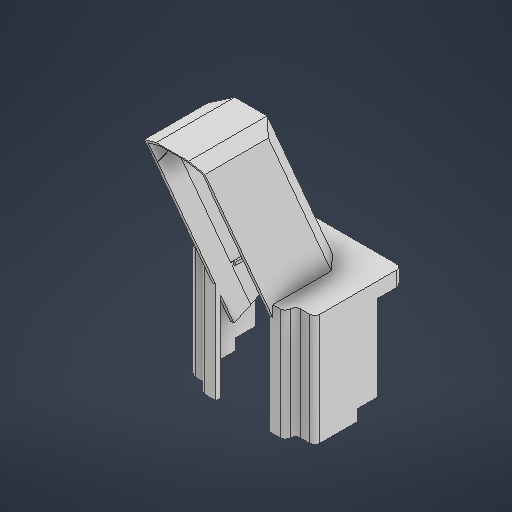
# Autodesk Inventor part: Cover^2 No magnets
Saved by Autodesk Inventor 2025 (Build 290162000, 162)
## iProperties
Created: 2025-02-14
Part Number: Cover^2 No magnets
Material: Generic
Document SubType Name: Modeling
Designer: mayhe
Density: 1 g/cm^3
Appearance: Default
Author: mayhe
Autodesk Inventor part; units mm, degrees
ref_plane "YZ Plane" through (0, 0, 0) normal (1, 0, 0) x (0, 1, 0)
ref_plane "XZ Plane" through (0, 0, 0) normal (0, 1, 0) x (-1, 0, 0)
ref_plane "XY Plane" through (0, 0, 0) normal (0, 0, 1) x (1, 0, 0)
sketch "Sketch1" plane through (0, 0, 0) normal (0, 1, 0) x (-1, 0, 0)
  line L0 (58.5, -37.5625) -> (-58.5, -37.5625)
  line L1 (-58.5, -37.5625) -> (-58.5, 37.5625)
  line L2 (-58.5, 37.5625) -> (58.5, 37.5625)
  line L3 (58.5, 37.5625) -> (58.5, -37.5625)
  line L4 (58.5, -37.5625) -> (-58.5, 37.5625) construction
  line L5 (-58.5, -37.5625) -> (58.5, 37.5625) construction
  line L6 (-61.5, -40.5625) -> (61.5, -40.5625)
  line L7 (61.5, -40.5625) -> (61.5, 37.5625)
  line L8 (-61.5, 37.5625) -> (-61.5, -40.5625)
  line L9 (-58.5, 37.5625) -> (-61.5, 37.5625)
  line L10 (58.5, 37.5625) -> (61.5, 37.5625)
  line L11 (-25, 25.0625) -> (25, 25.0625)
  line L12 (25, 25.0625) -> (25, 50.0625)
  line L13 (25, 50.0625) -> (-25, 50.0625)
  line L14 (-25, 50.0625) -> (-25, 25.0625)
  line L15 (-25, 25.0625) -> (25, 50.0625) construction
  line L16 (25, 25.0625) -> (-25, 50.0625) construction
  line L17 (61.5, 37.5625) -> (26.5, 37.5625)
  line L18 (26.5, 37.5625) -> (26.5, 52.5625)
  line L19 (-61.5, 37.5625) -> (-26.5, 37.5625)
  line L20 (-26.5, 37.5625) -> (-26.5, 52.5625)
  line L21 (25, 25.0625) -> (-25, 25.0625)
  line L22 (-25, 25.0625) -> (-25, 10.0625)
  line L23 (-25, 10.0625) -> (25, 10.0625)
  line L24 (25, 10.0625) -> (25, 25.0625)
  circle A0 centre (0, 10.0625) radius 25
  line L25 (61.5, 37.5625) -> (61.5, 45.5625)
  line L26 (61.5, 45.5625) -> (42.25, 45.5625)
  line L27 (42.25, 45.5625) -> (42.25, 55.5625)
  line L28 (42.25, 55.5625) -> (26.5, 55.5625)
  line L29 (26.5, 55.5625) -> (26.5, 52.5625)
  line L30 (-26.5, 52.5625) -> (-26.5, 55.5625)
  line L31 (-26.5, 55.5625) -> (-42.25, 55.5625)
  line L32 (-42.25, 55.5625) -> (-42.25, 45.5625)
  line L33 (-42.25, 45.5625) -> (-61.5, 45.5625)
  line L34 (-61.5, 45.5625) -> (-61.5, 37.5625)
  point P0 (0, 0)
  point P1 (0, 37.5625)
  point P2 (25, 37.5625)
  point P3 (-25, 37.5625)
  point P4 (-26.5, 37.5625)
  point P5 (26.5, 37.5625)
  point P6 (58.5, 37.5625)
  dimension "d1" = 75.125
  dimension "d2" = 3
  dimension "d10" = 50
  dimension "d11" = 25
  dimension "d23" = 3
  dimension "d33" = 50
  dimension "d34" = 15
  dimension "d65" = 8
  dimension "d67" = 10
  dimension "d69" = 15.75
  dimension "d70" = 10
  dimension "d71" = 19.25
  dimension "d72" = 8
  dimension "d85" = 15.75
  dimension "d86" = 19.25
  constraints: 70 end point, 14 perpendicular, 7 parallel, 6 horizontal, 6 midpoint, 1 point on line, 1 vertical, 3 other
  measures "d1" distance between parallel lines of L2 L0
  measures "d2" distance between parallel lines of L0 L6
  measures "d10" distance of L13.end L12.end
  measures "d11" distance of L12.end L11.end
  measures "d23" distance between parallel lines of L3 L7
  measures "d33" distance of L23.end L22.end
  measures "d34" distance of L22.end L21.end
  measures "d65" distance of L7.end L25.end
  measures "d67" distance of L26.end L27.end
  measures "d69" distance of L30.end L31.end
  measures "d70" distance of L31.end L32.end
  measures "d71" distance of L32.end L33.end
  measures "d72" distance of L33.end L8.start
  measures "d85" distance of L27.end L28.end
  measures "d86" distance of L25.end L26.end
extrude "Extrusion1" add sketch "Sketch1" along normal blind 3 contours L3 L10 L7 L6 L8 L9 L1 L0 | L0 L1 L2 L14 L22 A0 L24 L12 L3 | L2 L18 L29 L28 L27 L26 L25 L10 | L9 L34 L33 L32 L31 L30 L20 L2
sketch "Sketch2" plane through (0, 0, 0) normal (0, -1, 0) x (1, 0, 0)
  line L0 (-59.5, 43.5625) -> (-59.5, 20.5625)
  line L1 (-59.5, 20.5625) -> (-61.5, 20.5625)
  line L2 (-61.5, 20.5625) -> (-61.5, 45.5625)
  line L3 (0, 0) -> (0, 37.5625)
  line L4 (59.5, 20.5625) -> (61.5, 20.5625)
  line L5 (-42.25, 55.5625) -> (-26.5, 55.5625)
  line L6 (-26.5, 55.5625) -> (-26.5, 50.5625)
  line L7 (-26.5, 50.5625) -> (-40.25, 50.5625)
  line L8 (-42.25, 45.5625) -> (-61.5, 45.5625)
  line L9 (-59.5, 43.5625) -> (-40.25, 43.5625)
  line L10 (-40.25, 43.5625) -> (-40.25, 50.5625)
  line L11 (-42.25, 45.5625) -> (-42.25, 55.5625) projected
  line L12 (-42.25, 55.5625) -> (-42.25, 45.5625)
  line L13 (59.5, 43.5625) -> (59.5, 20.5625)
  line L14 (59.5, 20.5625) -> (61.5, 20.5625)
  line L15 (61.5, 20.5625) -> (61.5, 45.5625)
  line L16 (42.25, 55.5625) -> (26.5, 55.5625)
  line L17 (26.5, 55.5625) -> (26.5, 50.5625)
  line L18 (26.5, 50.5625) -> (40.25, 50.5625)
  line L19 (42.25, 45.5625) -> (61.5, 45.5625)
  line L20 (59.5, 43.5625) -> (40.25, 43.5625)
  line L21 (40.25, 43.5625) -> (40.25, 50.5625)
  line L22 (42.25, 45.5625) -> (42.25, 55.5625)
  line L23 (42.25, 55.5625) -> (42.25, 45.5625)
  point P0 (0, 25.0625)
  point P1 (-59.5, 53.5625)
  dimension "d6" = 2
  dimension "d27" = 5
  dimension "d76" = 2
  dimension "d77" = 2
  dimension "d78" = 19.25
  dimension "d79" = 19.25
  dimension "d80" = 25
  constraints: 46 end point, 11 symmetric about line, 4 perpendicular, 2 parallel, 1 coincident, 1 collinear, 1 horizontal, 1 vertical, 1 vertical alignment
  measures "d6" distance of L0.end L1.end
  measures "d27" distance of L5.end L6.end
  measures "d76" distance between parallel lines of L11 L10
  measures "d77" distance between parallel lines of L9 L8
  measures "d78" distance of L8.start L2.end
  measures "d79" distance of L0.start L9.end
  measures "d80" distance of L1.end L2.end
extrude "Extrusion2" add sketch "Sketch2" along normal blind 107.5
sketch "Sketch3" plane through (0, 0, 0) normal (0, -1, 0) x (1, 0, 0)
  line L0 (61.5, -40.5625) -> (-61.5, -40.5625) projected
  line L1 (-61.5, -40.5625) -> (61.5, -40.5625)
  line L2 (61.5, -40.5625) -> (61.5, -16.5625)
  line L3 (61.5, -16.5625) -> (56, -16.5625)
  line L4 (56, -16.5625) -> (56, -37.5625)
  line L5 (-61.5, -16.5625) -> (-61.5, -40.5625)
  line L6 (-61.5, -16.5625) -> (-56, -16.5625)
  line L7 (-56, -16.5625) -> (-56, -37.5625)
  line L8 (-56, -37.5625) -> (56, -37.5625)
  line L9 (-59.5, 20.4625) -> (-59.5, -16.5625)
  line L10 (-59.5, -16.5625) -> (-61.5, -16.5625)
  line L11 (61.5, 20.5625) -> (61.5, 55.5625) projected
  line L12 (61.5, 20.5625) -> (59.5, 20.5625)
  line L13 (59.5, 20.5625) -> (59.5, -16.5625)
  line L14 (59.5, -16.5625) -> (61.5, -16.5625)
  line L15 (61.5, -16.5625) -> (61.5, 20.5625)
  line L16 (-61.5, -40.5625) -> (-61.5, 45.5625) projected
  line L17 (-61.5, 20.5625) -> (-61.5, -16.5625)
  line L18 (-61.5, -16.5625) -> (-61.5, -40.5625)
  line L19 (-61.5, 20.5625) -> (-59.5, 20.5625) projected
  line L20 (-61.5, 20.5625) -> (-59.5, 20.5625)
  line L21 (-59.5, 20.5625) -> (-59.5, 20.4625)
  point P0 (0, 0)
  dimension "d12" = 24
  dimension "d13" = 5.5
  dimension "d15" = 90
  dimension "d20" = 5.5
  dimension "d22" = 3
  dimension "d31" = 2
  dimension "d32" = 2
  constraints: 36 end point, 8 perpendicular, 3 collinear, 3 horizontal, 3 point on line, 2 parallel
  measures "d12" distance of L0.start L2.end
  measures "d13" distance of L2.end L3.end
  measures "d15" angle of L4 L3
  measures "d20" distance of L5.start L6.end
  measures "d22" distance between parallel lines of L0 L8
  measures "d31" distance of L9.end L10.end
  measures "d32" distance of L14.end L13.end
extrude "Extrusion3" add sketch "Sketch3" along normal blind 12
fillet "Fillet1" radius 5 16 edges at (56, -6, -37.5625) (-56, -6, -37.5625) (61.5, -4.5, -40.5625) (-61.5, -4.5, -40.5625) (61.5, -52.25, 45.5625) (42.25, -52.25, 45.5625) (42.25, -52.25, 55.5625) (-42.25, -52.25, 55.5625) (-61.5, -52.25, 45.5625) (-42.25, -52.25, 45.5625) (-59.5, -53.75, 43.5625) (-40.25, -53.75, 50.5625) (-40.25, -53.75, 43.5625) (40.25, -53.75, 50.5625) (40.25, -53.75, 43.5625) (59.5, -53.75, 43.5625)
chamfer "Chamfer1" distance 3.5 angle 45 2 edges at (-56, -6, -16.5625) (56, -6, -16.5625)
ref_plane "Work Plane1" through (-42.25, 3, 55.5625) normal (0, 0.9187912, 0.3947439) x (1, 0, 0)
sketch "Sketch4" plane through (-42.25, 3, 55.5625) normal (0, 0.9187912, 0.3947439) x (1, 0, 0)
  line L0 (15.25, 63.1227) -> (69.25, 63.1227)
  line L1 (69.25, 63.1227) -> (69.25, 13.7819)
  ellipse E0 centre (42.25, 41.805) end of major axis (67.25, 41.805) minor radius 22.9698 (67.25, 41.805) -> (17.25, 41.805) ccw
  line L2 (42.25, 41.805) -> (15.25, 63.1227) construction
  line L3 (42.25, 41.805) -> (69.25, 63.1227) construction
  line L4 (12.25, 53.6373) -> (12.25, -4.3627)
  line L5 (72.25, -4.3627) -> (72.25, 53.6373)
  line L6 (72.25, 53.6373) -> (12.25, 53.6373)
  line L7 (15.75, 13.7819) -> (15.25, 13.7819)
  line L8 (15.75, 13.7819) -> (15.75, -4.3627)
  line L9 (67.75, 16.5382) -> (67.75, 0)
  line L10 (69.25, 13.7819) -> (68.75, 13.7819)
  line L11 (68.75, 13.7819) -> (68.75, -4.3627)
  line L12 (12.25, -4.3627) -> (15.75, -4.3627)
  line L13 (68.75, -4.3627) -> (72.25, -4.3627)
  line L14 (15.25, 13.7819) -> (15.25, 63.1227)
  line L15 (12.25, 53.6373) -> (12.25, 67.1227)
  line L16 (12.25, 67.1227) -> (72.25, 67.1227)
  line L17 (72.25, 67.1227) -> (72.25, 53.6373)
  point P0 (42.25, 49.0766)
  point P1 (15.25, 53.6373)
  point P2 (69.25, 53.6373)
  point P3 (42.25, 53.6373)
  point P4 (42.25, 64.7748)
  point P5 (42.25, 67.1227)
  point P6 (42.25, 63.1227)
  dimension "d36" = 54
  dimension "d39" = 58
  dimension "d40" = 3.5
  dimension "d41" = 60
  dimension "d47" = 4
  dimension "d57" = 3
  constraints: 32 end point, 3 midpoint, 3 point on line, 2 vertical alignment, 11 other
  measures "d36" distance of L0.start L0.end
  measures "d39" distance between parallel lines of L6 L12
  measures "d40" distance between parallel lines of L8 L4
  measures "d41" distance of L5.start L4.end
  measures "d47" distance between parallel lines of L0 L16
  measures "d57" distance between parallel lines of L14 L4
extrude "Extrusion4" add sketch "Sketch4" along normal blind 135 and the other way blind 55.8 contours L14 L6 L15 L16 L17 L1 L0 E0 | E0 L0 | L14 L7 L8 L12 L4 L6 | L6 L5 L13 L11 L10 L1
chamfer "Chamfer3" distance 14 angle 45 4 edges at (-30, 78.2665, 14.8441) (30, 78.2665, 14.8441) (-27, 77.4771, 18.8585) (27, 77.4771, 18.8585)
sketch "Sketch9" plane through (0, -12, 0) normal (0, -1, 0) x (1, 0, 0)
  line L0 (0, 0) -> (0, 50)
  line L1 (-61.5, 20.5625) -> (-59.5, 20.5625) projected
  line L2 (-59.5, -16.5625) -> (-59.5, 20.5625) projected
  line L3 (-61.5, 20.5625) -> (-59.5, 20.5625)
  line L4 (-59.5, 20.5625) -> (-59.5, -16.5625)
  line L5 (-59.5, -16.5625) -> (-61.5, -16.5625)
  line L6 (-61.5, -16.5625) -> (-61.5, 20.5625)
  line L7 (61.5, 20.5625) -> (59.5, 20.5625)
  line L8 (59.5, -16.5625) -> (59.5, 20.5625)
  line L9 (61.5, 20.5625) -> (59.5, 20.5625)
  line L10 (59.5, 20.5625) -> (59.5, -16.5625)
  line L11 (59.5, -16.5625) -> (61.5, -16.5625)
  line L12 (61.5, -16.5625) -> (61.5, 20.5625)
  dimension "d92" = 50
  constraints: 22 end point, 5 symmetric about line, 2 parallel, 1 horizontal, 1 perpendicular, 1 vertical
  measures "d92" distance of L0.start L0.end
extrude "Extrusion8" add sketch "Sketch9" along normal blind 95.5
sketch "Sketch10" plane through (0, -107.5, 0) normal (0, -1, 0) x (1, 0, 0)
  line L0 (-59.5, -16.5625) -> (-56, -20.0625) projected
  line L1 (-61.5, 40.5625) -> (-61.5, -16.5625) projected
  line L2 (-59.5, -16.5625) -> (-61.5, -16.5625)
  line L3 (-61.5, -16.5625) -> (-61.5, 3.4375)
  line L4 (-61.5, 3.4375) -> (-59.5, 3.4375)
  line L5 (-59.5, 3.4375) -> (-59.5, -16.5625)
  line L6 (0, 0) -> (0, 17.4625)
  line L7 (59.5, -16.5625) -> (56, -20.0625)
  line L8 (61.5, 40.5625) -> (61.5, -16.5625)
  line L9 (59.5, -16.5625) -> (61.5, -16.5625)
  line L10 (61.5, -16.5625) -> (61.5, 3.4375)
  line L11 (61.5, 3.4375) -> (59.5, 3.4375)
  line L12 (59.5, 3.4375) -> (59.5, -16.5625)
  dimension "d93" = 20
  constraints: 22 end point, 7 symmetric about line, 2 parallel, 2 point on line, 1 horizontal, 1 perpendicular, 1 vertical
  measures "d93" distance of L2.end L3.end
extrude "Extrusion9" cut sketch "Sketch10" against normal blind 11
ref_plane "Work Plane5" through (-30, 64.798, 86.8613) normal (0, 0, 1) x (1, 0, 0)
sketch "Sketch13" plane through (-30, 64.798, 86.8613) normal (0, 0, 1) x (1, 0, 0)
  line L0 (46, 88.7351) -> (14, 88.7351)
  line L1 (14, 88.7351) -> (46, 88.7351)
  line L2 (60, 83.2086) -> (60, -61.798)
  line L3 (46, 88.7351) -> (60, 83.2086)
  line L4 (60, 83.2086) -> (60, 48.2086)
  line L5 (60, 48.2086) -> (57, 48.2086)
  line L6 (57, -61.798) -> (57, 81.6297)
  line L7 (57, 81.6297) -> (43, 87.1561)
  line L8 (17, 87.1561) -> (3, 81.6297)
  line L9 (43, 87.1561) -> (17, 87.1561)
  line L10 (17, 87.1561) -> (3, 81.6297)
  line L11 (3, 81.6297) -> (3, 48.2086)
  line L12 (3, 48.2086) -> (0, 48.2086)
  line L13 (0, -61.798) -> (0, 83.2086)
  line L14 (0, 83.2086) -> (14, 88.7351)
  point P0 (60, 48.2086)
  dimension "d117" = 35
  constraints: 30 end point, 3 parallel, 3 point on line, 2 collinear, 1 perpendicular
  measures "d117" distance of L2.start L4.end
extrude "Extrusion13" add sketch "Sketch13" against normal through all
extrude "Extrusion14" add sketch "Sketch13" along normal up to surface surface through (-30, 1.2779, 59.5709) normal (0, -0.3947439, 0.9187912)
body "Solid1"
